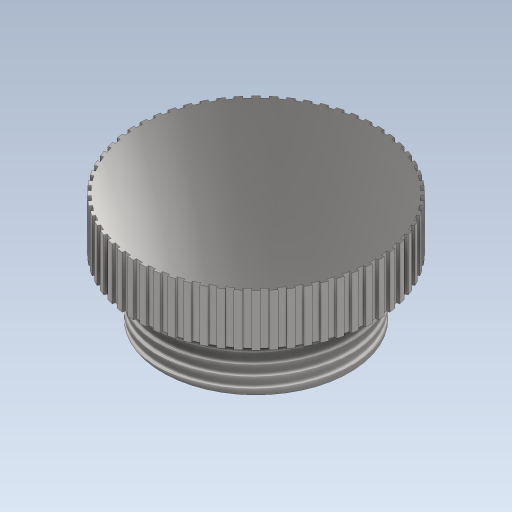
# Autodesk Inventor part: Pump-Motor-CW-Rotation:Cover 101
Saved by Autodesk Inventor 2024.2 (Build 282272000, 272)
## iProperties
Created: 2025-06-16
Material: Steel, Alloy
Document SubType Name: Modeling
Density: 7.73 g/cm^3
Appearance: Semi-Polished
Designer: cw
Author: cw
Autodesk Inventor part; units mm, degrees
ref_plane "YZ Plane" through (0, 0, 0) normal (1, 0, 0) x (0, 1, 0)
ref_plane "XZ Plane" through (0, 0, 0) normal (0, 1, 0) x (-1, 0, 0)
ref_plane "XY Plane" through (0, 0, 0) normal (0, 0, 1) x (1, 0, 0)
sketch "Sketch1" plane through (0, 0, 0) normal (0, 0, 1) x (1, 0, 0)
  circle A0 centre (0, 0) radius 23
  dimension "d0" = 46
  constraints: 1 centre point, 1 coincident
  measures "d0" diameter of A0
extrude "Extrusion1" add sketch "Sketch1" along normal blind 10
sketch "Sketch2" plane through (0, 0, 0) normal (0, 0, -1) x (-1, 0, 0)
  circle A0 centre (0, 0) radius 18
  dimension "d3" = 36
  constraints: 1 centre point, 1 coincident
  measures "d3" diameter of A0
extrude "Extrusion2" add sketch "Sketch2" along normal blind 11
sketch "Sketch3" plane through (0, 0, 10) normal (0, 0, 1) x (1, 0, 0)
  line L0 (0, 0) -> (-0.6021, 22.9921)
  circle A0 centre (0, 0) radius 23 projected
  line L1 (0, 0) -> (0.6021, 22.9921)
  arc A1 (0.589, 22.4923) -> (-0.589, 22.4923) centre (0, 0) ccw
  dimension "d6" = 22.5
  dimension "d7" = 3
  constraints: 4 end point, 4 point on circle, 2 point on line, 1 centre point, 1 coincident, 1 horizontal alignment
  measures "d6" radius of A1
  measures "d7" angle of L1 L0
extrude "Extrusion3" cut sketch "Sketch3" against normal through all contours L0 A0 L1 A1
pattern_circular "Circular Pattern1" count 60 over 360 about axis through (0, 0, -10) along (0, 0, 1) of "Extrusion3"
sketch "Sketch4" plane through (0, 0, -11) normal (0, 0, -1) x (-1, 0, 0)
  point P0 (0, 0)
hole "Hole1" at (0, 0, -11) direction (0, 0, 1) diameter 28 depth 11
thread "Thread1" size "M36x2" class "6g" standard "ISO Metric profile" full length
body "Solid1"
